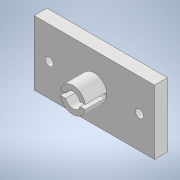
# Autodesk Inventor part: pin_1
Saved by Autodesk Inventor 2020 (Build 240168000, 168)
## iProperties
Created: 2020-05-02
Part Number: pin_1
Material: Generic
Document SubType Name: Modeling
Designer: psrobotics
Density: 1 g/cm^3
Appearance: Default
Author: psrobotics
Autodesk Inventor part; units mm, degrees
ref_plane "YZ Plane" through (0, 0, 0) normal (1, 0, 0) x (0, 1, 0)
ref_plane "XZ Plane" through (0, 0, 0) normal (0, 1, 0) x (-1, 0, 0)
ref_plane "XY Plane" through (0, 0, 0) normal (0, 0, 1) x (1, 0, 0)
sketch "Sketch1" plane through (0, 0, 0) normal (0, 0, 1) x (1, 0, 0)
  circle A0 centre (10.5, -1.5) radius 0.95 projected
  circle A1 centre (-10.5, -1.5) radius 0.95 projected
  line L0 (14, 9) -> (-14, 9) projected
  line L1 (-14, 9) -> (-14, -9) projected
  line L2 (-14, -9) -> (-7.5, -9) projected
  line L3 (-7.5, -9) -> (-7.5, -1.5) projected
  arc A2 (7.5, -1.5) -> (-7.5, -1.5) centre (0, -1.5) ccw projected
  line L4 (7.5, -1.5) -> (7.5, -9) projected
  line L5 (7.5, -9) -> (14, -9) projected
  line L6 (14, -9) -> (14, 9) projected
  line L7 (-7.5, -9) -> (7.5, -9)
  point P0 (0, 0)
  constraints: 2 end point, 1 collinear
extrude "Extrusion1" add sketch "Sketch1" along normal blind 3
sketch "Sketch2" plane through (0, 0, 3) normal (0, 0, 1) x (1, 0, 0)
  circle A0 centre (0, -1.5) radius 3 projected
  circle A1 centre (0, -1.5) radius 2.95
  point P0 (0, 0)
  dimension "d4" = 5.9
  constraints: 1 centre point, 1 coincident
  measures "d4" diameter of A1
extrude "Extrusion2" add sketch "Sketch2" along normal blind 5 contours A1
sketch "Sketch3" plane through (0, -1.5, 8) normal (0, 0, 1) x (1, 0, 0)
  circle A0 centre (0, 0) radius 2.95 projected
  circle A1 centre (0, 0) radius 1.75
  point P0 (0, 1.5)
  dimension "d7" = 3.5
  constraints: 1 centre point, 1 coincident
  measures "d7" diameter of A1
extrude "Extrusion3" cut sketch "Sketch3" against normal blind 8 contours A1
sketch "Sketch4" plane through (0, 0, 3) normal (0, 0, 1) x (1, 0, 0)
  circle A0 centre (0, -1.5) radius 2.95 projected
  line L0 (14, -9) -> (14, 9) projected
  line L1 (14, 9) -> (-14, 9) projected
  line L2 (-14, 9) -> (-14, -9) projected
  line L3 (-14, -9) -> (14, -9) projected
  circle A1 centre (10.5, -1.5) radius 0.95 projected
  circle A2 centre (-10.5, -1.5) radius 0.95 projected
  line L4 (-5, -2) -> (-5, -1)
  line L5 (-5, -1) -> (5, -1)
  line L6 (5, -1) -> (5, -2)
  line L7 (5, -2) -> (-5, -2)
  line L8 (-5, -2) -> (5, -1) construction
  line L9 (-5, -1) -> (5, -2) construction
  point P0 (0, 0)
  dimension "d10" = 1
  dimension "d11" = 10
  constraints: 12 end point, 2 midpoint, 2 parallel, 1 perpendicular, 1 vertical
  measures "d10" distance of L4.start L4.end
  measures "d11" distance of L4.end L5.end
extrude "Extrusion4" cut sketch "Sketch4" along normal up to surface (5 mm away) contours A0 L7 L5 | A0 L5 L6 L7 | A0 L7 L4 L5
fillet "Fillet1" radius 0.5 4 edges at (-2.2922, -2, 3) (-2.2922, -1, 3) (2.2922, -2, 3) (2.2922, -1, 3)
sketch "Sketch5" plane through (0, 0, 3) normal (0, 0, 1) x (1, 0, 0)
  arc A0 (2.95, -1.5) -> (-2.95, -1.5) centre (0, -1.5) ccw projected
  arc A1 (-2.95, -1.5) -> (2.95, -1.5) centre (0, -1.5) ccw projected
  line L0 (14, -9) -> (14, 9) projected
  line L1 (14, 9) -> (-14, 9) projected
  line L2 (-14, 9) -> (-14, -9) projected
  line L3 (-14, -9) -> (14, -9) projected
  circle A2 centre (10.5, -1.5) radius 0.95 projected
  circle A3 centre (-10.5, -1.5) radius 0.95 projected
  line L4 (-17.5, -6.5) -> (-17.5, 3.5)
  line L5 (-17.5, 3.5) -> (17.5, 3.5)
  line L6 (17.5, 3.5) -> (17.5, -6.5)
  line L7 (17.5, -6.5) -> (-17.5, -6.5)
  line L8 (-17.5, -6.5) -> (17.5, 3.5) construction
  line L9 (-17.5, 3.5) -> (17.5, -6.5) construction
  point P0 (0, 0)
  point P1 (-14, 3.5)
  point P2 (14, 3.5)
  point P3 (14, -6.5)
  point P4 (-14, -6.5)
  dimension "d15" = 10
  dimension "d16" = 35
  constraints: 12 end point, 2 midpoint, 2 parallel, 1 perpendicular, 1 vertical
  measures "d15" distance of L4.start L4.end
  measures "d16" distance of L4.end L5.end
extrude "Extrusion5" cut sketch "Sketch5" against normal blind 8 contours L3 L2 L7 L0 | L5 L2 L1 L0
chamfer "Chamfer1" distance 2 angle 45 4 edges at (-14, 3.5, 1.5) (-14, -6.5, 1.5) (14, 3.5, 1.5) (14, -6.5, 1.5)
body "Solid1"
